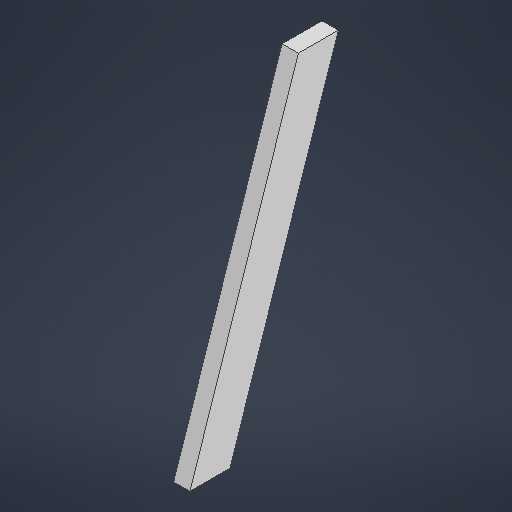
# Autodesk Inventor part: taildiag
Saved by Autodesk Inventor 2027.1 (Build 311270010, 270A)
## iProperties
Created: 2026-09-04
Part Number: taildiag
Material: Generic
Document SubType Name: Modeling
Designer: jorda
Density: 1 g/cm^3
Appearance: Default
Author: jorda
Autodesk Inventor part; units mm, degrees
ref_plane "YZ Plane" through (0, 0, 0) normal (1, 0, 0) x (0, 1, 0)
ref_plane "XZ Plane" through (0, 0, 0) normal (0, 1, 0) x (-1, 0, 0)
ref_plane "XY Plane" through (0, 0, 0) normal (0, 0, 1) x (1, 0, 0)
sketch "Sketch1" plane through (0, 0, 0) normal (1, 0, 0) x (0, 1, 0)
  line L0 (0, -93.7088) -> (0, 0)
  line L1 (0, 0) -> (761.2673, -253.7558)
  line L2 (760.9969, -347.3745) -> (633.2735, -304.8)
  line L3 (633.2735, -304.8) -> (0, -93.7088)
  line L4 (761.2673, -253.7558) -> (760.9969, -347.3745)
  constraints: 10 end point
extrude "Extrusion1" add sketch "Sketch1" along normal blind 38.1
body "Solid1"
